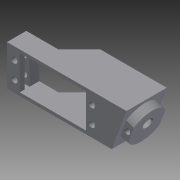
# Autodesk Inventor part: forearm
Saved by Autodesk Inventor 2015 (Build 190159000, 159)
## iProperties
Created: 2015-09-26
Part Number: forearm
Material: Générique
Document SubType Name: Modeling
Designer: astralien3000
Density: 1 g/cm^3
Appearance: Par défaut
Author: astralien3000
Autodesk Inventor part; units mm, degrees
ref_plane "YZ Plane" through (0, 0, 0) normal (1, 0, 0) x (0, 1, 0)
ref_plane "XZ Plane" through (0, 0, 0) normal (0, 1, 0) x (-1, 0, 0)
ref_plane "XY Plane" through (0, 0, 0) normal (0, 0, 1) x (1, 0, 0)
sketch "Esquisse1" plane through (0, 0, 0) normal (0, 1, 0) x (-1, 0, 0)
  line L0 (20.5, 10.5) -> (-20.5, 10.5)
  line L1 (-20.5, 10.5) -> (-20.5, -10.5)
  line L2 (-20.5, -10.5) -> (20.5, -10.5)
  line L3 (20.5, -10.5) -> (20.5, 10.5)
  line L4 (28.5, 12.5) -> (-36.5, 12.5)
  line L5 (-36.5, 12.5) -> (-36.5, -12.5)
  line L6 (-36.5, -12.5) -> (28.5, -12.5)
  line L7 (28.5, -12.5) -> (28.5, 12.5)
  line L8 (-36.5, -12.5) -> (-45.5993, 12.5)
  line L9 (-45.5993, 12.5) -> (-36.5, 12.5)
  point P0 (0, 0)
  dimension "d0" = 20
  dimension "d1" = 41
  dimension "d2" = 21
  dimension "d3" = 10.5
  dimension "d4" = 20.5
  dimension "d5" = 8
  dimension "d6" = 2
  dimension "d7" = 2
  dimension "d8" = 16
  constraints: 20 end point, 4 parallel, 2 horizontal, 2 perpendicular, 1 collinear
  measures "d0" angle of L5 L8
  measures "d1" distance of L1.end L2.end
  measures "d2" distance of L2.end L0.start
  measures "d3" distance from line of L2 point (0, 0)
  measures "d4" distance from line of L1 point (0, 0)
  measures "d5" distance between parallel lines of L7 L3
  measures "d6" distance between parallel lines of L0 L4
  measures "d7" distance between parallel lines of L6 L2
  measures "d8" distance between parallel lines of L1 L5
extrude "Extrusion1" add sketch "Esquisse1" along normal mid plane 25
sketch "Esquisse2" plane through (36.5, -12.5, -12.5) normal (0.9397, 0, -0.342) x (-0.342, 0, -0.9397)
  line L0 (-26.6044, 25) -> (0, 0)
  line L1 (0, 0) -> (0, 25)
  line L2 (0, 25) -> (-26.6044, 0)
  arc A0 (-8.3022, 22.298) -> (-18.3022, 22.298) centre (-13.3022, 12.5) ccw
  line L3 (-18.3022, 22.298) -> (-8.3022, 22.298)
  line L4 (-8.3022, 22.298) -> (-8.3022, 2.702)
  line L5 (-8.3022, 2.702) -> (-18.3022, 2.702)
  line L6 (-18.3022, 2.702) -> (-18.3022, 22.298)
  arc A1 (-8.3022, 2.702) -> (-8.3022, 22.298) centre (-13.3022, 12.5) ccw
  arc A2 (-18.3022, 2.702) -> (-8.3022, 2.702) centre (-13.3022, 12.5) ccw
  arc A3 (-18.3022, 22.298) -> (-18.3022, 2.702) centre (-13.3022, 12.5) ccw
  point P0 (0.7376, 12.5)
  dimension "d11" = 22
  dimension "d13" = 10
  constraints: 14 end point, 9 point on circle, 4 centre point, 4 coincident, 2 parallel, 1 horizontal, 1 midpoint, 1 perpendicular, 1 vertical
  measures "d11" diameter of A0
  measures "d13" distance of L3.start L3.end
extrude "Extrusion2" add sketch "Esquisse2" along normal blind 5 contours A3 L6 L0 | L0 L6 L2 A3 | L6 L3 L4 L2 L0 | L0 L2 L6 | L2 L6 A3 | L2 L4 L0 | L0 L4 L5 L6 L2 | A1 L2 L4 | L4 L2 A1 L0 | L0 A1 L4
sketch "Esquisse3" plane through (39.3395, -9.798, -4.6985) normal (0, -1, 0) x (0.9397, 0, -0.342)
  line L0 (5, 10) -> (0, 0)
  line L1 (0, 10) -> (5, 0)
  circle A0 centre (2.5, 5) radius 1.75
  point P0 (-38.574, -9.0398)
  dimension "d16" = 3.5
  constraints: 4 end point, 1 centre point, 1 coincident, 1 midpoint
  measures "d16" diameter of A0
extrude "Extrusion3" cut sketch "Esquisse3" against normal through all
sketch "Esquisse4" plane through (20.5, -12.5, 10.5) normal (-1, 0, 0) x (0, 0, 1)
  line L0 (-21, 3) -> (0, 3)
  line L1 (0, 3) -> (0, 6)
  line L2 (0, 6) -> (-21, 6)
  line L3 (-21, 6) -> (-21, 3)
  line L4 (-21, 0) -> (-21, 25) projected
  line L5 (0, 0) -> (0, 25) projected
  line L6 (0, 0) -> (-21, 0) projected
  point P0 (-10.5, 12.5)
  dimension "d19" = 3
  dimension "d20" = 3
  constraints: 8 end point, 2 collinear, 2 parallel, 1 horizontal, 1 perpendicular, 1 other
  measures "d19" distance of the line from the sketch origin of L0
  measures "d20" distance between parallel lines of L0 L2
extrude "Extrusion4" cut sketch "Esquisse4" against normal blind 7 contours L3 L2 L1 L0
sketch "Esquisse5" plane through (-20.5, -12.5, -10.5) normal (1, 0, 0) x (0, 0, -1)
  line L0 (-21, 6) -> (0, 6)
  line L1 (0, 6) -> (0, 3)
  line L2 (0, 3) -> (-21, 3)
  line L3 (-21, 3) -> (-21, 6)
  line L4 (-21, 25) -> (-21, 0) projected
  line L5 (0, 0) -> (0, 25) projected
  line L6 (0, 0) -> (-21, 0) projected
  point P0 (-10.5, 12.5)
  dimension "d23" = 3
  dimension "d24" = 3
  constraints: 8 end point, 2 collinear, 2 parallel, 1 horizontal, 1 perpendicular, 1 other
  measures "d23" distance of the line from the sketch origin of L2
  measures "d24" distance between parallel lines of L2 L0
extrude "Extrusion5" cut sketch "Esquisse5" against normal blind 7 contours L0 L1 L2 L3
sketch "Esquisse6" plane through (20.5, 12.5, -10.5) normal (-1, 0, 0) x (0, 0, 1)
  line L0 (21, -25) -> (0, 0)
  line L1 (0, -25) -> (21, 0)
  circle A0 centre (10.5, -12.5) radius 3
  dimension "d27" = 6
  constraints: 4 end point, 2 coincident, 1 centre point
  measures "d27" diameter of A0
extrude "Extrusion6" cut sketch "Esquisse6" against normal through all
sketch "Esquisse7" plane through (20.5, 12.5, -10.5) normal (-1, 0, 0) x (0, 0, 1)
  circle A0 centre (10.5, -12.5) radius 3
  circle A1 centre (10.5, -12.5) radius 1.75
  circle A2 centre (10.5, -12.5) radius 3 projected
  dimension "d30" = 0
  dimension "d31" = 3.5
  constraints: 2 centre point, 2 coincident
  measures "d30" radial gap between concentric circles of A0 A2
  measures "d31" diameter of A1
extrude "Extrusion7" add sketch "Esquisse7" against normal blind 18
sketch "Esquisse8" plane through (20.5, 12.5, -10.5) normal (-1, 0, 0) x (0, 0, 1)
  circle A0 centre (10.5, -12.5) radius 3
  dimension "d34" = 6
  constraints: 1 centre point, 1 coincident
  measures "d34" diameter of A0
extrude "Extrusion8" cut sketch "Esquisse8" against normal blind 3
sketch "Esquisse10" plane through (0, -12.5, 0) normal (0, -1, 0) x (1, 0, 0)
  line L0 (-20.5, -10.5) -> (-27.5, -10.5)
  line L1 (-27.5, -10.5) -> (-27.5, 10.5)
  line L2 (-27.5, 10.5) -> (-20.5, 10.5)
  line L3 (-20.5, 10.5) -> (-20.5, -10.5)
  line L4 (20.5, -10.5) -> (27.5, -10.5)
  line L5 (27.5, -10.5) -> (27.5, 10.5)
  line L6 (27.5, 10.5) -> (20.5, 10.5)
  line L7 (20.5, 10.5) -> (20.5, -10.5)
  line L8 (-27.5, -10.5) -> (-27.5, 10.5) projected
  line L9 (27.5, 10.5) -> (27.5, -10.5) projected
  line L10 (-27.5, -10.5) -> (-20.5, 0)
  line L11 (-20.5, 0) -> (-27.5, 10.5)
  line L12 (-27.5, 0) -> (-20.5, 10.5)
  line L13 (-20.5, -10.5) -> (-27.5, 0)
  line L14 (20.5, -10.5) -> (27.5, 0)
  line L15 (20.5, 0) -> (27.5, -10.5)
  line L16 (27.5, 10.5) -> (20.5, 0)
  line L17 (20.5, 10.5) -> (27.5, 0)
  circle A0 centre (-24, -5.25) radius 2
  circle A1 centre (24, -5.25) radius 2
  circle A2 centre (24, 5.25) radius 2
  circle A3 centre (-24, 5.25) radius 2
  point P0 (0, 0)
  dimension "d37" = 4
  dimension "d38" = 4
  dimension "d39" = 4
  dimension "d40" = 4
  constraints: 32 end point, 8 midpoint, 6 parallel, 4 centre point, 2 coincident, 2 collinear, 2 horizontal, 2 perpendicular
  measures "d37" diameter of A3
  measures "d38" diameter of A0
  measures "d39" diameter of A2
  measures "d40" diameter of A1
extrude "Extrusion9" cut sketch "Esquisse10" against normal through all contours A0 L10 L13 | L13 L10 A0 | A0 L13 L10 | L10 L13 A0 | A3 L12 L11 | L11 L12 A3 | A3 L11 L12 | L12 L11 A3 | A1 L15 L14 | L14 L15 A1 | L15 L14 A1 | A1 L14 L15 | A2 L17 L16 | L16 L17 A2 | L17 L16 A2 | A2 L16 L17
sketch "Esquisse11" plane through (36.5, 12.5, -12.5) normal (0, 0, -1) x (-1, 0, 0)
  line L0 (65, 0) -> (45, 0)
  line L1 (45, 0) -> (45, -13)
  line L2 (45, -13) -> (65, -13)
  line L3 (65, -13) -> (65, 0)
  line L4 (65, -25) -> (0, -25) projected
  line L5 (45, -13) -> (32, 0)
  line L6 (0, 0) -> (65, 0) projected
  line L7 (45, 0) -> (32, 0)
  point P0 (36.5, -12.5)
  dimension "d43" = 20
  dimension "d44" = 12
  dimension "d45" = 45
  constraints: 12 end point, 2 horizontal, 2 parallel, 1 perpendicular, 1 point on line
  measures "d43" distance of L1.end L2.end
  measures "d44" distance between parallel lines of L2 L4
  measures "d45" angle of L1 L5
extrude "Extrusion10" cut sketch "Esquisse11" against normal through all
equation "\"d3\" = 0.5 * d2"
equation "\"d4\" = 0.5 * d1"
equation "\"d38\" = d37"
equation "\"d39\" = d37"
equation "\"d40\" = d37"
